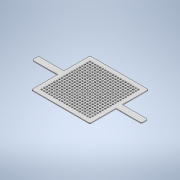
# Autodesk Inventor part: MouldCover20x20
Saved by Autodesk Inventor 2020.3 (Build 243373010, 373A)
## iProperties
Created: 2020-10-26
Part Number: MouldCover20x20
Material: Generic
Document SubType Name: Modeling
Designer: Naude Conradie
Density: 1 g/cm^3
Appearance: Default
Author: Naude Conradie
Autodesk Inventor part; units mm, degrees
ref_plane "YZ Plane" through (0, 0, 0) normal (1, 0, 0) x (0, 1, 0)
ref_plane "XZ Plane" through (0, 0, 0) normal (0, 1, 0) x (-1, 0, 0)
ref_plane "XY Plane" through (0, 0, 0) normal (0, 0, 1) x (1, 0, 0)
sketch "Sketch1" plane through (0, 0, 0) normal (0, 1, 0) x (-1, 0, 0)
  line L0 (0, 0) -> (230, 0)
  line L1 (230, 0) -> (230, -230)
  line L2 (230, -230) -> (0, -230)
  line L3 (0, -230) -> (0, 0)
  dimension "d0" = 230
  dimension "d1" = 230
  constraints: 8 end point, 2 parallel, 1 horizontal, 1 perpendicular
  measures "d0" distance of L1.end L2.end
  measures "d1" distance of L0.end L1.end
extrude "Extrusion1" add sketch "Sketch1" along normal blind 3
sketch "Sketch2" plane through (0, 3, 0) normal (0, 1, 0) x (1, 0, 0)
  line L0 (-230, 0) -> (0, 0) projected
  line L1 (0, 0) -> (0, 230) projected
  point P0 (-20, 20)
  point P1 (-30, 20)
  point P2 (-40, 20)
  point P3 (-50, 20)
  point P4 (-60, 20)
  point P5 (-70, 20)
  point P6 (-80, 20)
  point P7 (-90, 20)
  point P8 (-100, 20)
  point P9 (-110, 20)
  point P10 (-120, 20)
  point P11 (-130, 20)
  point P12 (-140, 20)
  point P13 (-150, 20)
  point P14 (-160, 20)
  point P15 (-170, 20)
  point P16 (-180, 20)
  point P17 (-190, 20)
  point P18 (-200, 20)
  point P19 (-210, 20)
  point P20 (-20, 30)
  point P21 (-30, 30)
  point P22 (-40, 30)
  point P23 (-50, 30)
  point P24 (-60, 30)
  point P25 (-70, 30)
  point P26 (-80, 30)
  point P27 (-90, 30)
  point P28 (-100, 30)
  point P29 (-110, 30)
  point P30 (-120, 30)
  point P31 (-130, 30)
  point P32 (-140, 30)
  point P33 (-150, 30)
  point P34 (-160, 30)
  point P35 (-170, 30)
  point P36 (-180, 30)
  point P37 (-190, 30)
  point P38 (-200, 30)
  point P39 (-210, 30)
  point P40 (-20, 40)
  point P41 (-30, 40)
  point P42 (-40, 40)
  point P43 (-50, 40)
  point P44 (-60, 40)
  point P45 (-70, 40)
  point P46 (-80, 40)
  point P47 (-90, 40)
  point P48 (-100, 40)
  point P49 (-110, 40)
  point P50 (-120, 40)
  point P51 (-130, 40)
  point P52 (-140, 40)
  point P53 (-150, 40)
  point P54 (-160, 40)
  point P55 (-170, 40)
  point P56 (-180, 40)
  point P57 (-190, 40)
  point P58 (-200, 40)
  point P59 (-210, 40)
  point P60 (-20, 50)
  point P61 (-30, 50)
  point P62 (-40, 50)
  point P63 (-50, 50)
  point P64 (-60, 50)
  point P65 (-70, 50)
  point P66 (-80, 50)
  point P67 (-90, 50)
  point P68 (-100, 50)
  point P69 (-110, 50)
  point P70 (-120, 50)
  point P71 (-130, 50)
  point P72 (-140, 50)
  point P73 (-150, 50)
  point P74 (-160, 50)
  point P75 (-170, 50)
  point P76 (-180, 50)
  point P77 (-190, 50)
  point P78 (-200, 50)
  point P79 (-210, 50)
  point P80 (-20, 60)
  point P81 (-30, 60)
  point P82 (-40, 60)
  point P83 (-50, 60)
  point P84 (-60, 60)
  point P85 (-70, 60)
  point P86 (-80, 60)
  point P87 (-90, 60)
  point P88 (-100, 60)
  point P89 (-110, 60)
  point P90 (-120, 60)
  point P91 (-130, 60)
  point P92 (-140, 60)
  point P93 (-150, 60)
  point P94 (-160, 60)
  point P95 (-170, 60)
  point P96 (-180, 60)
  point P97 (-190, 60)
  point P98 (-200, 60)
  point P99 (-210, 60)
  point P100 (-20, 70)
  point P101 (-30, 70)
  point P102 (-40, 70)
  point P103 (-50, 70)
  point P104 (-60, 70)
  point P105 (-70, 70)
  point P106 (-80, 70)
  point P107 (-90, 70)
  point P108 (-100, 70)
  point P109 (-110, 70)
  point P110 (-120, 70)
  point P111 (-130, 70)
  point P112 (-140, 70)
  point P113 (-150, 70)
  point P114 (-160, 70)
  point P115 (-170, 70)
  point P116 (-180, 70)
  point P117 (-190, 70)
  point P118 (-200, 70)
  point P119 (-210, 70)
  point P120 (-20, 80)
  point P121 (-30, 80)
  point P122 (-40, 80)
  point P123 (-50, 80)
  point P124 (-60, 80)
  point P125 (-70, 80)
  point P126 (-80, 80)
  point P127 (-90, 80)
  point P128 (-100, 80)
  point P129 (-110, 80)
  point P130 (-120, 80)
  point P131 (-130, 80)
  point P132 (-140, 80)
  point P133 (-150, 80)
  point P134 (-160, 80)
  point P135 (-170, 80)
  point P136 (-180, 80)
  point P137 (-190, 80)
  point P138 (-200, 80)
  point P139 (-210, 80)
  point P140 (-20, 90)
  point P141 (-30, 90)
  point P142 (-40, 90)
  point P143 (-50, 90)
  point P144 (-60, 90)
  point P145 (-70, 90)
  point P146 (-80, 90)
  point P147 (-90, 90)
  point P148 (-100, 90)
  point P149 (-110, 90)
  point P150 (-120, 90)
  point P151 (-130, 90)
  point P152 (-140, 90)
  point P153 (-150, 90)
  point P154 (-160, 90)
  point P155 (-170, 90)
  point P156 (-180, 90)
  point P157 (-190, 90)
  point P158 (-200, 90)
  point P159 (-210, 90)
  point P160 (-20, 100)
  point P161 (-30, 100)
  point P162 (-40, 100)
  point P163 (-50, 100)
  point P164 (-60, 100)
  point P165 (-70, 100)
  point P166 (-80, 100)
  point P167 (-90, 100)
  point P168 (-100, 100)
  point P169 (-110, 100)
  point P170 (-120, 100)
  point P171 (-130, 100)
  point P172 (-140, 100)
  point P173 (-150, 100)
  point P174 (-160, 100)
  point P175 (-170, 100)
  point P176 (-180, 100)
  point P177 (-190, 100)
  point P178 (-200, 100)
  point P179 (-210, 100)
  point P180 (-20, 110)
  point P181 (-30, 110)
  point P182 (-40, 110)
  point P183 (-50, 110)
  point P184 (-60, 110)
  point P185 (-70, 110)
  point P186 (-80, 110)
  point P187 (-90, 110)
  point P188 (-100, 110)
  point P189 (-110, 110)
  point P190 (-120, 110)
  point P191 (-130, 110)
  point P192 (-140, 110)
  point P193 (-150, 110)
  point P194 (-160, 110)
  point P195 (-170, 110)
  point P196 (-180, 110)
  point P197 (-190, 110)
  point P198 (-200, 110)
  point P199 (-210, 110)
  dimension "d4" = 20
  dimension "d5" = 20
  dimension "d8" = 10
  dimension "d11" = 10
  constraints: 1 horizontal, 1 vertical, 399 other
  measures "d4" distance from line of L0 point (-20, 20)
  measures "d5" distance from line of L1 point (-20, 20)
  measures "d8" distance of point (-20, 20) point (-30, 20)
  measures "d11" distance of point (-20, 20) point (-20, 30)
hole "Hole1" at (-20, 3, -20) at (-30, 3, -20) at (-40, 3, -20) at (-50, 3, -20) at (-60, 3, -20) at (-70, 3, -20) at (-80, 3, -20) at (-90, 3, -20) at (-100, 3, -20) at (-110, 3, -20) at (-120, 3, -20) at (-130, 3, -20) at (-140, 3, -20) at (-150, 3, -20) at (-160, 3, -20) at (-170, 3, -20) at (-180, 3, -20) at (-190, 3, -20) at (-200, 3, -20) at (-210, 3, -20) at (-20, 3, -30) at (-30, 3, -30) at (-40, 3, -30) at (-50, 3, -30) at (-60, 3, -30) at (-70, 3, -30) at (-80, 3, -30) at (-90, 3, -30) at (-100, 3, -30) at (-110, 3, -30) at (-120, 3, -30) at (-130, 3, -30) at (-140, 3, -30) at (-150, 3, -30) at (-160, 3, -30) at (-170, 3, -30) at (-180, 3, -30) at (-190, 3, -30) at (-200, 3, -30) at (-210, 3, -30) at (-20, 3, -40) at (-30, 3, -40) at (-40, 3, -40) at (-50, 3, -40) at (-60, 3, -40) at (-70, 3, -40) at (-80, 3, -40) at (-90, 3, -40) at (-100, 3, -40) at (-110, 3, -40) direction (0, -1, 0) diameter 6 end through all and at (-120, 3, -40) (-130, 3, -40) (-140, 3, -40) (-150, 3, -40) (-160, 3, -40) (-170, 3, -40) (-180, 3, -40) (-190, 3, -40) (-200, 3, -40) (-210, 3, -40) (-20, 3, -50) (-30, 3, -50) (-40, 3, -50) (-50, 3, -50) (-60, 3, -50) (-70, 3, -50) (-80, 3, -50) (-90, 3, -50) (-100, 3, -50) (-110, 3, -50) (-120, 3, -50) (-130, 3, -50) (-140, 3, -50) (-150, 3, -50) (-160, 3, -50) (-170, 3, -50) (-180, 3, -50) (-190, 3, -50) (-200, 3, -50) (-210, 3, -50) (-20, 3, -60) (-30, 3, -60) (-40, 3, -60) (-50, 3, -60) (-60, 3, -60) (-70, 3, -60) (-80, 3, -60) (-90, 3, -60) (-100, 3, -60) (-110, 3, -60) (-120, 3, -60) (-130, 3, -60) (-140, 3, -60) (-150, 3, -60) (-160, 3, -60) (-170, 3, -60) (-180, 3, -60) (-190, 3, -60) (-200, 3, -60) (-210, 3, -60) (-20, 3, -70) (-30, 3, -70) (-40, 3, -70) (-50, 3, -70) (-60, 3, -70) (-70, 3, -70) (-80, 3, -70) (-90, 3, -70) (-100, 3, -70) (-110, 3, -70) (-120, 3, -70) (-130, 3, -70) (-140, 3, -70) (-150, 3, -70) (-160, 3, -70) (-170, 3, -70) (-180, 3, -70) (-190, 3, -70) (-200, 3, -70) (-210, 3, -70) (-20, 3, -80) (-30, 3, -80) (-40, 3, -80) (-50, 3, -80) (-60, 3, -80) (-70, 3, -80) (-80, 3, -80) (-90, 3, -80) (-100, 3, -80) (-110, 3, -80) (-120, 3, -80) (-130, 3, -80) (-140, 3, -80) (-150, 3, -80) (-160, 3, -80) (-170, 3, -80) (-180, 3, -80) (-190, 3, -80) (-200, 3, -80) (-210, 3, -80) (-20, 3, -90) (-30, 3, -90) (-40, 3, -90) (-50, 3, -90) (-60, 3, -90) (-70, 3, -90) (-80, 3, -90) (-90, 3, -90) (-100, 3, -90) (-110, 3, -90) (-120, 3, -90) (-130, 3, -90) (-140, 3, -90) (-150, 3, -90) (-160, 3, -90) (-170, 3, -90) (-180, 3, -90) (-190, 3, -90) (-200, 3, -90) (-210, 3, -90) (-20, 3, -100) (-30, 3, -100) (-40, 3, -100) (-50, 3, -100) (-60, 3, -100) (-70, 3, -100) (-80, 3, -100) (-90, 3, -100) (-100, 3, -100) (-110, 3, -100) (-120, 3, -100) (-130, 3, -100) (-140, 3, -100) (-150, 3, -100) (-160, 3, -100) (-170, 3, -100) (-180, 3, -100) (-190, 3, -100) (-200, 3, -100) (-210, 3, -100) (-20, 3, -110) (-30, 3, -110) (-40, 3, -110) (-50, 3, -110) (-60, 3, -110) (-70, 3, -110) (-80, 3, -110) (-90, 3, -110) (-100, 3, -110) (-110, 3, -110) (-120, 3, -110) (-130, 3, -110) (-140, 3, -110) (-150, 3, -110) (-160, 3, -110) (-170, 3, -110) (-180, 3, -110) (-190, 3, -110) (-200, 3, -110) (-210, 3, -110) (-20, 3, -120) (-30, 3, -120) (-40, 3, -120) (-50, 3, -120) (-60, 3, -120) (-70, 3, -120) (-80, 3, -120) (-90, 3, -120) (-100, 3, -120) (-110, 3, -120) (-120, 3, -120) (-130, 3, -120) (-140, 3, -120) (-150, 3, -120) (-160, 3, -120) (-170, 3, -120) (-180, 3, -120) (-190, 3, -120) (-200, 3, -120) (-210, 3, -120) (-20, 3, -130) (-30, 3, -130) (-40, 3, -130) (-50, 3, -130) (-60, 3, -130) (-70, 3, -130) (-80, 3, -130) (-90, 3, -130) (-100, 3, -130) (-110, 3, -130) (-120, 3, -130) (-130, 3, -130) (-140, 3, -130) (-150, 3, -130) (-160, 3, -130) (-170, 3, -130) (-180, 3, -130) (-190, 3, -130) (-200, 3, -130) (-210, 3, -130) (-20, 3, -140) (-30, 3, -140) (-40, 3, -140) (-50, 3, -140) (-60, 3, -140) (-70, 3, -140) (-80, 3, -140) (-90, 3, -140) (-100, 3, -140) (-110, 3, -140) (-120, 3, -140) (-130, 3, -140) (-140, 3, -140) (-150, 3, -140) (-160, 3, -140) (-170, 3, -140) (-180, 3, -140) (-190, 3, -140) (-200, 3, -140) (-210, 3, -140) (-20, 3, -150) (-30, 3, -150) (-40, 3, -150) (-50, 3, -150) (-60, 3, -150) (-70, 3, -150) (-80, 3, -150) (-90, 3, -150) (-100, 3, -150) (-110, 3, -150) (-120, 3, -150) (-130, 3, -150) (-140, 3, -150) (-150, 3, -150) (-160, 3, -150) (-170, 3, -150) (-180, 3, -150) (-190, 3, -150) (-200, 3, -150) (-210, 3, -150) (-20, 3, -160) (-30, 3, -160) (-40, 3, -160) (-50, 3, -160) (-60, 3, -160) (-70, 3, -160) (-80, 3, -160) (-90, 3, -160) (-100, 3, -160) (-110, 3, -160) (-120, 3, -160) (-130, 3, -160) (-140, 3, -160) (-150, 3, -160) (-160, 3, -160) (-170, 3, -160) (-180, 3, -160) (-190, 3, -160) (-200, 3, -160) (-210, 3, -160) (-20, 3, -170) (-30, 3, -170) (-40, 3, -170) (-50, 3, -170) (-60, 3, -170) (-70, 3, -170) (-80, 3, -170) (-90, 3, -170) (-100, 3, -170) (-110, 3, -170) (-120, 3, -170) (-130, 3, -170) (-140, 3, -170) (-150, 3, -170) (-160, 3, -170) (-170, 3, -170) (-180, 3, -170) (-190, 3, -170) (-200, 3, -170) (-210, 3, -170) (-20, 3, -180) (-30, 3, -180) (-40, 3, -180) (-50, 3, -180) (-60, 3, -180) (-70, 3, -180) (-80, 3, -180) (-90, 3, -180) (-100, 3, -180) (-110, 3, -180) (-120, 3, -180) (-130, 3, -180) (-140, 3, -180) (-150, 3, -180) (-160, 3, -180) (-170, 3, -180) (-180, 3, -180) (-190, 3, -180) (-200, 3, -180) (-210, 3, -180) (-20, 3, -190) (-30, 3, -190) (-40, 3, -190) (-50, 3, -190) (-60, 3, -190) (-70, 3, -190) (-80, 3, -190) (-90, 3, -190) (-100, 3, -190) (-110, 3, -190) (-120, 3, -190) (-130, 3, -190) (-140, 3, -190) (-150, 3, -190) (-160, 3, -190) (-170, 3, -190) (-180, 3, -190) (-190, 3, -190) (-200, 3, -190) (-210, 3, -190) (-20, 3, -200) (-30, 3, -200) (-40, 3, -200) (-50, 3, -200) (-60, 3, -200) (-70, 3, -200) (-80, 3, -200) (-90, 3, -200) (-100, 3, -200) (-110, 3, -200) (-120, 3, -200) (-130, 3, -200) (-140, 3, -200) (-150, 3, -200) (-160, 3, -200) (-170, 3, -200) (-180, 3, -200) (-190, 3, -200) (-200, 3, -200) (-210, 3, -200) (-20, 3, -210) (-30, 3, -210) (-40, 3, -210) (-50, 3, -210) (-60, 3, -210) (-70, 3, -210) (-80, 3, -210) (-90, 3, -210) (-100, 3, -210) (-110, 3, -210) (-120, 3, -210) (-130, 3, -210) (-140, 3, -210) (-150, 3, -210) (-160, 3, -210) (-170, 3, -210) (-180, 3, -210) (-190, 3, -210) (-200, 3, -210) (-210, 3, -210)
chamfer "Chamfer1" distance 2 angle 45 4 edges at (-230, 1.5, -230) (0, 1.5, -230) (0, 1.5, 0) (-230, 1.5, 0)
sketch "Sketch3" plane through (0, 0, -2) normal (1, 0, 0) x (0, 0, -1)
  line L0 (100.5, 0) -> (125.5, 0)
  line L1 (125.5, 0) -> (125.5, 3)
  line L2 (125.5, 3) -> (100.5, 3)
  line L3 (100.5, 3) -> (100.5, 0)
  point P0 (-2, 0)
  dimension "d24" = 25
  dimension "d25" = 102.5
  constraints: 8 end point, 2 parallel, 1 horizontal, 1 perpendicular
  measures "d24" distance of L2.end L1.end
  measures "d25" distance of point (-2, 0) L0.start
extrude "Extrusion2" add sketch "Sketch3" along normal blind 100
sketch "Sketch4" plane through (-230, 0, -228) normal (-1, 0, 0) x (0, 0, 1)
  line L0 (0, 3) -> (226, 3) projected
  line L1 (100.5, 0) -> (0, 0) projected
  line L2 (100.5, 0) -> (125.5, 0)
  line L3 (125.5, 0) -> (125.5, 3)
  line L4 (125.5, 3) -> (100.5, 3)
  line L5 (100.5, 3) -> (100.5, 0)
  line L6 (-2, 3) -> (-2, 0) projected
  point P0 (228, 0)
  dimension "d28" = 25
  dimension "d29" = 102.5
  constraints: 8 end point, 2 parallel, 2 point on line, 1 horizontal, 1 perpendicular
  measures "d28" distance of L4.end L3.end
  measures "d29" distance from line of L6 L2.start
extrude "Extrusion3" add sketch "Sketch4" along normal blind 100
chamfer "Chamfer2" distance 5 angle 45 4 edges at (-330, 1.5, -102.5) (-330, 1.5, -127.5) (100, 1.5, -102.5) (100, 1.5, -127.5)
body "Solid1"
